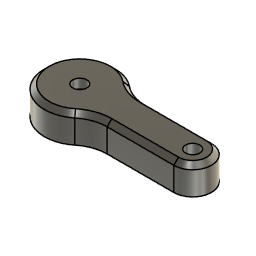
Smart_Gripper (Autodesk Fusion 360 archive; units mm, degrees)
design "servo_arm"
Autodesk Fusion 360 part; units mm, degrees
sketch "Sketch1" plane through (0, 0, 0) normal (0, 0, 1) x (1, 0, 0)
  circle A0 centre (0, 0) radius 7.5
  line L0 (0, 4) -> (28, 4)
  line L1 (28, 4) -> (28, -4)
  line L2 (28, -4) -> (0, -4)
  line L3 (0, -4) -> (0, 4)
  circle A1 centre (0, 0) radius 1.5
  circle A2 centre (24, 0) radius 1.5
  dimension "d1" = 15
  dimension "d2" = 28
  dimension "d3" = 8
  dimension "d4" = 4
  dimension "d5" = 3
  dimension "d6" = 3
  dimension "d7" = 24
  constraint coincident A0.centre A1.centre
  constraint horizontal L0
  constraint vertical L1
  constraint horizontal L2
  constraint vertical L3
  measures "d1" diameter of A0
  measures "d2" distance of L0.start L0.end
  measures "d3" distance of L0.end L1.end
  measures "d4" distance of A0.centre L0
  measures "d5" diameter of A1
  measures "d6" diameter of A2
  measures "d7" distance of A0.centre A2.centre
extrude "Extrude1" add sketch "Sketch1" along normal blind 6 contours A0 L0 L2 L3 A1 | A0 L0 L1 L2 | A0 L0 L2 L3 A1
fillet "Fillet1" radius 8 2 edges at (6.3443, -4, 3) (6.3443, 4, 3)
fillet "Fillet2" radius 4 2 edges at (28, 4, 3) (28, -4, 3)
chamfer "Chamfer1" distance 1 angle 45 6 edges at (16.9054, -4, 6) (28, 0, 6) (16.9054, 4, 6) (7.1226, 4.4651, 6) (-7.5, 0, 6) (7.1226, -4.4651, 6)
sketch "Sketch2" plane through (0, 0, 0) normal (0, 0, -1) x (1, 0, 0)
  arc A0 (24, -4) -> (24, 4) centre (24, 0) ccw
  line L0 (24, 4) -> (9.8107, 4)
  arc A1 (4.7471, 5.8065) -> (9.8107, 4) centre (9.8107, 12) ccw
  arc A2 (4.7471, 5.8065) -> (4.7471, -5.8065) centre (0, 0) ccw
  arc A3 (9.8107, -4) -> (4.7471, -5.8065) centre (9.8107, -12) ccw
  line L1 (9.8107, -4) -> (24, -4)
  circle A4 centre (24, 0) radius 1.5
  circle A5 centre (0, 0) radius 1.5
  circle A6 centre (0, 0) radius 3
  dimension "d15" = 6
  constraint coincident A2.centre A5.centre
  measures "d15" diameter of A6
extrude "Extrude2" cut sketch "Sketch2" against normal blind 4 contours A6
